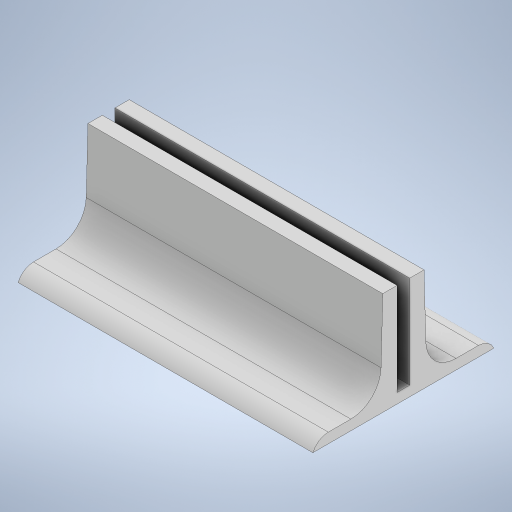
# Autodesk Inventor part: cleat bracket v1
Saved by Autodesk Inventor 2024 (Build 280153020, 153B)
## iProperties
Created: 2024-02-13
Part Number: cleat bracket v1
Material: Generic
Document SubType Name: Modeling
Designer: scottst
Density: 1 g/cm^3
Appearance: Default
Author: scottst
Autodesk Inventor part; units mm, degrees
ref_plane "YZ Plane" through (0, 0, 0) normal (1, 0, 0) x (0, 1, 0)
ref_plane "XZ Plane" through (0, 0, 0) normal (0, 1, 0) x (-1, 0, 0)
ref_plane "XY Plane" through (0, 0, 0) normal (0, 0, 1) x (1, 0, 0)
sketch "Sketch1" plane through (0, 0, 0) normal (1, 0, 0) x (0, 1, 0)
  line L0 (0, 0) -> (0, -0.75) construction
  line L1 (0, 0) -> (0, 0.75) construction
  line L2 (0, 0.75) -> (11, 0.75)
  line L3 (11, 0.75) -> (11, 2.45)
  line L4 (0, -0.75) -> (11, -0.75)
  line L5 (11, -0.75) -> (11, -2.45)
  line L6 (0, 0.75) -> (0, 2.75)
  line L7 (0, 2.75) -> (11, 2.45)
  line L8 (0, -0.75) -> (0, -2.75)
  line L9 (0, -2.75) -> (11, -2.45)
  line L10 (0, -0.75) -> (0, 0.75)
  line L11 (0, 2.75) -> (0, 10.75)
  line L12 (0, -2.75) -> (0, -10.75)
  line L13 (0, -2.75) -> (8, -2.75) construction
  line L14 (0, -10.75) -> (-1.2, -10.75)
  line L15 (-1.2, -10.75) -> (-1.2, 10.75)
  line L16 (-1.2, 10.75) -> (0, 10.75)
  dimension "d0" = 0.75
  dimension "d1" = 0.75
  dimension "d2" = 11
  dimension "d3" = 1.7
  dimension "d4" = 11
  dimension "d5" = 1.7
  dimension "d6" = 2
  dimension "d7" = 2
  dimension "d8" = 8
  dimension "d9" = 8
  dimension "d10" = 90
  dimension "d11" = 1.2
  constraints: 34 end point, 7 vertical, 4 perpendicular, 3 horizontal, 1 collinear, 1 parallel
  measures "d0" distance of L0.start L0.end
  measures "d1" distance of L0.start L1.end
  measures "d2" distance of L1.end L2.end
  measures "d3" distance of L2.end L3.end
  measures "d4" distance of L0.end L4.end
  measures "d5" distance of L4.end L5.end
  measures "d6" distance of L1.end L6.end
  measures "d7" distance of L0.end L8.end
  measures "d8" distance of L6.end L11.end
  measures "d9" distance of L8.end L12.end
  measures "d10" angle of L12 L13
  measures "d11" distance of L12.end L14.end
extrude "Extrusion1" add sketch "Sketch1" along normal blind 35
fillet "Fillet1" radius 3.5875 2 edges at (17.5, 0, 2.75) (17.5, 0, -2.75)
fillet "Fillet2" radius 2 2 edges at (17.5, 0, 10.75) (17.5, 0, -10.75)
body "Solid1"
